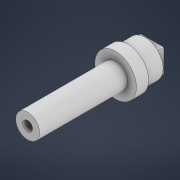
# Autodesk Inventor part: Welle_Kugellager_Mitte
Saved by Autodesk Inventor 2021 (Build 250183000, 183)
## iProperties
Created: 2021-01-30
Part Number: Welle_Kugellager_Mitte
Material: Generisch
Document SubType Name: Modeling
Designer: Ctroi
Density: 1 g/cm^3
Appearance: Vorgabe
Author: Ctroi
Autodesk Inventor part; units mm, degrees
ref_plane "YZ Plane" through (0, 0, 0) normal (1, 0, 0) x (0, 1, 0)
ref_plane "XZ Plane" through (0, 0, 0) normal (0, 1, 0) x (-1, 0, 0)
ref_plane "XY Plane" through (0, 0, 0) normal (0, 0, 1) x (1, 0, 0)
sketch "Skizze1" plane through (0, 0, 0) normal (0, 0, 1) x (1, 0, 0)
  line L0 (-4.75, 4.75) -> (4.75, 4.75)
  line L1 (4.75, 4.75) -> (4.75, -4.75)
  line L2 (4.75, -4.75) -> (-4.75, -4.75)
  line L3 (-4.75, -4.75) -> (-4.75, 4.75)
  line L4 (-4.75, 4.75) -> (4.75, -4.75) construction
  line L5 (4.75, 4.75) -> (-4.75, -4.75) construction
  point P0 (0, 0)
  dimension "d0" = 9.5
  dimension "d1" = 9.5
  constraints: 12 end point, 2 midpoint, 2 parallel, 1 horizontal, 1 perpendicular
  measures "d0" distance of L1.end L2.end
  measures "d1" distance of L0.end L1.end
extrude "Extrusion1" add sketch "Skizze1" along normal blind 3
sketch "Skizze2" plane through (0, 0, 3) normal (0, 0, 1) x (1, 0, 0)
  circle A0 centre (0, 0) radius 7.4
  dimension "d4" = 14.8
  constraints: 1 centre point, 1 coincident
  measures "d4" diameter of A0
extrude "Extrusion2" add sketch "Skizze2" along normal blind 7
sketch "Skizze5" plane through (0, 0, 0) normal (0, 0, -1) x (-1, 0, 0)
  circle A0 centre (0, 0) radius 2
  dimension "d13" = 4
  constraints: 1 centre point, 1 coincident
  measures "d13" diameter of A0
extrude "Extrusion5" cut sketch "Skizze5" against normal blind 5
sketch "Skizze6" plane through (0, 0, 10) normal (0, 0, 1) x (1, 0, 0)
  circle A0 centre (0, 0) radius 8.5
  dimension "d16" = 17
  constraints: 1 centre point, 1 coincident
  measures "d16" diameter of A0
extrude "Extrusion6" add sketch "Skizze6" along normal blind 5
sketch "Skizze7" plane through (0, 0, 15) normal (0, 0, 1) x (1, 0, 0)
  circle A0 centre (0, 0) radius 4.9
  dimension "d19" = 9.8
  constraints: 1 centre point, 1 coincident
  measures "d19" diameter of A0
extrude "Extrusion7" add sketch "Skizze7" along normal blind 36
sketch "Skizze8" plane through (0, 0, 51) normal (0, 0, 1) x (1, 0, 0)
  circle A0 centre (0, 0) radius 2
  dimension "d22" = 4
  constraints: 1 centre point, 1 coincident
  measures "d22" diameter of A0
extrude "Extrusion8" cut sketch "Skizze8" against normal blind 5
